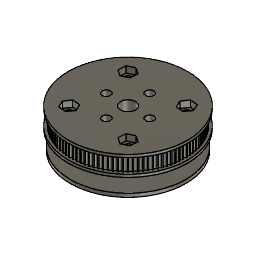
çark1 (Autodesk Fusion 360 design; units mm, degrees)
Autodesk Fusion 360 part; units mm, degrees
sketch "Sketch1" plane through (0, 0, 0) normal (0, 0, 1) x (1, 0, 0)
  circle A0 centre (0, 0) radius 4.1
  circle A1 centre (0, 0) radius 32
  dimension "d1" = 8.2
  dimension "d2" = 64
  constraint coincident A0.centre A1.centre
  measures "d1" diameter of A0
  measures "d2" diameter of A1
extrude "Extrude1" add sketch "Sketch1" along normal blind 2
sketch "Sketch3" plane through (0, 0, 2) normal (0, 0, 1) x (-1, 0, 0)
  circle A0 centre (0, 0) radius 4.1
  circle A1 centre (0, 0) radius 32
  circle A2 centre (0, 0) radius 12.5
  circle A3 centre (0, 0) radius 4.1
  dimension "d5" = 25
  dimension "d6" = 8.2
  constraint coincident A0.centre A1.centre
  measures "d5" diameter of A2
  measures "d6" diameter of A3
extrude "Extrude2" add sketch "Sketch3" along normal blind 9.8 contours A2
sketch "Sketch4" plane through (0, 0, 11.8) normal (0, 0, 1) x (-1, 0, 0)
  circle A0 centre (0, 0) radius 4.1
  circle A1 centre (0, 0) radius 12.5
  circle A2 centre (0, 0) radius 4.1
  circle A3 centre (0, 0) radius 31.575
  dimension "d9" = 8.2
  dimension "d10" = 63.15
  constraint coincident A0.centre A1.centre
  measures "d9" diameter of A2
  measures "d10" diameter of A3
extrude "Extrude3" add sketch "Sketch4" along normal blind 8 contours A1 | A3
sketch "Sketch5" plane through (0, 0, 19.8) normal (0, 0, 1) x (-1, 0, 0)
  circle A0 centre (0, 0) radius 4.1
  circle A1 centre (0, 0) radius 31.575
  line L0 (0, 0) -> (0, 32)
  circle A2 centre (0, 32) radius 0.7
  dimension "d13" = 1.4
  constraint coincident A0.centre A1.centre
  constraint vertical L0
  constraint coincident L0.end A2.centre
  measures "d13" diameter of A2
sketch "Sketch7" plane through (0, 0, 19.8) normal (0, 0, 1) x (-1, 0, 0)
  circle A0 centre (0, 0) radius 4.1
  circle A1 centre (0, 0) radius 31.575
  circle A2 centre (0, 0) radius 4.1
  circle A3 centre (0, 0) radius 33
  dimension "d21" = 66
  constraint coincident A0.centre A1.centre
  constraint concentric A2 A3
  measures "d21" diameter of A3
extrude "Extrude6" add sketch "Sketch7" along normal blind 1.5 contours A1 | A3
sketch "Sketch8" plane through (0, 0, 11.8) normal (0, 0, -1) x (1, 0, 0)
  circle A0 centre (0, 0) radius 31.575
  circle A1 centre (0, 0) radius 12.5
  circle A2 centre (0, 0) radius 33
  dimension "d24" = 66
  constraint concentric A0 A2
  measures "d24" diameter of A2
extrude "Extrude7" add sketch "Sketch8" along normal blind 1.5 contours A0 | A2
sketch "Sketch9" plane through (0, 0, 21.3) normal (0, 0, 1) x (-1, 0, 0)
  circle A0 centre (0, 0) radius 4.1
  circle A1 centre (0, 0) radius 33
  circle A2 centre (0, 0) radius 31.575
  line L0 (0, 0) -> (0, -38)
  circle A3 centre (0, -31.573) radius 0.7
  dimension "d27" = 63.15
  dimension "d28" = 1.4
  constraint concentric A0 A2
  constraint coincident A0.centre A1.centre
  constraint vertical L0
  constraint coincident L0 A3.centre
  measures "d27" diameter of A2
  measures "d28" diameter of A3
extrude "Extrude8" cut sketch "Sketch9" against normal blind 8 from surface at -1.5 contours A2 L0 A3 | A2 L0 A3 picked at (-0.1432, -31.3501) picked at (0.1432, -31.3501)
pattern_circular "C-Pattern2" count 100 over 360 about axis through (0, 0, 0) along (0, 0, 1) of "Extrude8"
sketch "Sketch10" plane through (0, 0, 21.3) normal (0, 0, 1) x (-1, 0, 0)
  circle A0 centre (0, 0) radius 4.1
  circle A1 centre (0, 0) radius 33
  circle A2 centre (0, 0) radius 12
  circle A3 centre (0, 0) radius 23
  line L0 (0, 0) -> (0, -36.5764)
  line L1 (0, 0) -> (-29, -29)
  circle A4 centre (0, -12) radius 2.25
  circle A5 centre (-16.2635, -16.2635) radius 2.25
  line L2 (-20.4072, -15.9325) -> (-18.6219, -19.6865)
  line L3 (-18.6219, -19.6865) -> (-14.4782, -20.0175)
  line L4 (-14.4782, -20.0175) -> (-12.1197, -16.5944)
  line L5 (-12.1197, -16.5944) -> (-13.905, -12.8404)
  line L6 (-13.905, -12.8404) -> (-18.0487, -12.5094)
  line L7 (-18.0487, -12.5094) -> (-20.4072, -15.9325)
  circle A6 centre (16.2635, -16.2635) radius 2.25
  line L8 (15.9325, -20.4072) -> (19.6865, -18.6219)
  line L9 (19.6865, -18.6219) -> (20.0175, -14.4782)
  line L10 (20.0175, -14.4782) -> (16.5944, -12.1197)
  line L11 (16.5944, -12.1197) -> (12.8404, -13.905)
  line L12 (12.8404, -13.905) -> (12.5094, -18.0487)
  line L13 (12.5094, -18.0487) -> (15.9325, -20.4072)
  circle A7 centre (12, 0) radius 2.25
  circle A8 centre (16.2635, 16.2635) radius 2.25
  line L14 (20.4072, 15.9325) -> (18.6219, 19.6865)
  line L15 (18.6219, 19.6865) -> (14.4782, 20.0175)
  line L16 (14.4782, 20.0175) -> (12.1197, 16.5944)
  line L17 (12.1197, 16.5944) -> (13.905, 12.8404)
  line L18 (13.905, 12.8404) -> (18.0487, 12.5094)
  line L19 (18.0487, 12.5094) -> (20.4072, 15.9325)
  circle A9 centre (0, 12) radius 2.25
  circle A10 centre (-16.2635, 16.2635) radius 2.25
  line L20 (-15.9325, 20.4072) -> (-19.6865, 18.6219)
  line L21 (-19.6865, 18.6219) -> (-20.0175, 14.4782)
  line L22 (-20.0175, 14.4782) -> (-16.5944, 12.1197)
  line L23 (-16.5944, 12.1197) -> (-12.8404, 13.905)
  line L24 (-12.8404, 13.905) -> (-12.5094, 18.0487)
  line L25 (-12.5094, 18.0487) -> (-15.9325, 20.4072)
  circle A11 centre (-12, 0) radius 2.25
  point P0 (-16.2635, -16.2635)
  dimension "d34" = 24
  dimension "d35" = 46
  dimension "d36" = 4.5
  dimension "d37" = 4.5
  dimension "d38" = 3.6
  dimension "d40" = 360
  constraint coincident A0.centre A1.centre
  constraint concentric A0 A3
  constraint vertical L0
  constraint coincident A2 A4.centre
  constraint coincident L0 A4.centre
  constraint coincident A3 P0
  constraint coincident L1 P0
  constraint coincident P0 A5.centre
  measures "d34" diameter of A2
  measures "d35" diameter of A3
  measures "d36" diameter of A4
  measures "d37" diameter of A5
  measures "d38" distance of P0 L7
extrude "Extrude9" cut sketch "Sketch10" against normal blind 15 contours A2 L0 A4 | A2 L0 A4 | A2 A11 | A2 A11 | A2 L0 A4 | A2 L0 A4 | A3 L1 A5 | A3 L1 A5 | A2 A7 | A2 A7 | A2 A9 | A2 A9 | A3 L1 A5 | A3 L1 A5 | A3 A6 | A3 A6 | A3 A10 | A3 A10 | A3 A8 | A3 A8
extrude "Extrude10" cut sketch "Sketch10" against normal blind 3.5 contours A3 L1 A5 L4 L5 | A3 L1 A5 L5 L6 L7 | A3 L1 A5 L2 L7 | A3 L1 A5 L2 L3 L4 | A3 A6 L10 L11 L12 L13 | A3 A6 L8 L9 L10 L13 | A3 A10 L20 L21 L22 L25 | A3 A10 L22 L23 L24 L25 | A3 A8 L16 L17 L18 L19 | A3 A8 L14 L15 L16 L19
